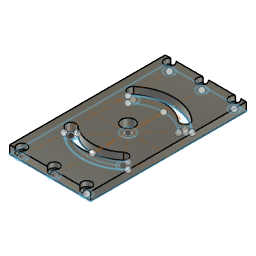
FS80 Pivot Base v3 (Autodesk Fusion 360 design; units mm, degrees)
Autodesk Fusion 360 part; units mm, degrees
sketch "Schizzo5" plane through (0, 0, 0) normal (0, 0, 1) x (1, 0, 0)
  line L0 (80.7173, 86.3147) -> (80.7173, -9.6853)
  circle A0 centre (85.7173, -7.1853) radius 1.5
  circle A1 centre (105.7173, 38.3147) radius 25 construction
  arc A2 (125.5163, 58.1137) -> (105.7173, 66.3147) centre (105.7173, 38.3147) ccw
  circle A3 centre (121.787, 57.4658) radius 3
  circle A4 centre (89.6476, 57.4658) radius 3
  arc A5 (105.7173, 66.3147) -> (85.9183, 58.1137) centre (105.7173, 38.3147) ccw
  circle A6 centre (125.7173, 83.8147) radius 3
  arc A7 (105.7173, 10.3147) -> (125.5163, 18.5157) centre (105.7173, 38.3147) ccw
  line L1 (80.7173, 38.3147) -> (130.7173, 38.3147) construction
  circle A8 centre (105.7173, 83.8147) radius 1.5
  circle A9 centre (85.7173, 83.8147) radius 3
  line L2 (105.7173, 38.3147) -> (121.787, 19.1636) construction
  arc A10 (105.7173, 66.3147) -> (85.9183, 58.1137) centre (105.7173, 38.3147) ccw
  circle A11 centre (85.7173, 83.8147) radius 1.5
  line L3 (130.7173, 86.3147) -> (80.7173, 86.3147)
  arc A12 (125.5163, 58.1137) -> (105.7173, 66.3147) centre (105.7173, 38.3147) ccw
  circle A13 centre (125.7173, 83.8147) radius 1.5
  line L4 (105.7173, 38.3147) -> (89.6274, 54.4047) construction
  circle A14 centre (105.7173, 83.8147) radius 3
  arc A15 (105.7173, 10.3147) -> (125.5163, 18.5157) centre (105.7173, 38.3147) ccw
  line L5 (105.7173, 38.3147) -> (105.7173, 13.3147) construction
  circle A16 centre (105.7173, 38.3147) radius 4.1
  circle A17 centre (105.7173, -7.1853) radius 1.5
  circle A18 centre (89.6476, 19.1636) radius 3
  line L6 (130.7173, -9.6853) -> (130.7173, 86.3147)
  arc A19 (85.9183, 18.5157) -> (105.7173, 10.3147) centre (105.7173, 38.3147) ccw
  line L7 (85.7173, 86.3147) -> (85.7173, -9.6853) construction
  arc A20 (105.7173, 13.3147) -> (121.787, 19.1636) centre (105.7173, 38.3147) ccw
  circle A21 centre (121.787, 19.1636) radius 3
  circle A22 centre (85.7173, -7.1853) radius 3
  circle A23 centre (105.7173, -7.1853) radius 3
  circle A24 centre (125.7173, -7.1853) radius 1.5
  line L8 (105.7173, 38.3147) -> (123.668, 56.2654) construction
  line L9 (80.7173, -9.6853) -> (130.7173, -9.6853)
  circle A25 centre (125.7173, -7.1853) radius 3
  line L10 (80.7173, -7.1853) -> (130.7173, -7.1853) construction
  line L11 (105.7173, 38.3147) -> (89.6476, 19.1636) construction
  arc A26 (85.9183, 18.5157) -> (105.7173, 10.3147) centre (105.7173, 38.3147) ccw
  line L12 (105.7173, 86.3147) -> (105.7173, -9.6853) construction
  arc A27 (89.6476, 19.1636) -> (105.7173, 13.3147) centre (105.7173, 38.3147) ccw
  line L13 (105.7173, 38.3147) -> (105.7173, 63.3147) construction
  line L14 (105.7173, 38.3147) -> (105.7173, 63.3147) construction
  line L15 (105.7173, 38.3147) -> (105.7173, 13.3147) construction
  arc A28 (105.7173, 16.3147) -> (121.2737, 22.7584) centre (105.7173, 38.3147) ccw
  arc A29 (90.161, 22.7584) -> (105.7173, 16.3147) centre (105.7173, 38.3147) ccw
  arc A30 (105.7173, 60.3147) -> (90.161, 53.8711) centre (105.7173, 38.3147) ccw
  arc A31 (121.2737, 53.8711) -> (105.7173, 60.3147) centre (105.7173, 38.3147) ccw
  dimension "d219" = 3
  dimension "d220" = 3
  dimension "d221" = 50
  dimension "d222" = 96
  dimension "d223" = 2.5
  dimension "d224" = 20
  dimension "d225" = 3
  dimension "d226" = 6
  dimension "d227" = 3
  dimension "d228" = 6
  dimension "d229" = 8.2
  dimension "d230" = 40
  dimension "d231" = 6
  dimension "d232" = 40
  dimension "d233" = 6
  dimension "d246" = -3
  dimension "d247" = -3
  constraint horizontal L9
  constraint vertical L6
  constraint horizontal L3
  constraint vertical L0
  constraint midpoint L12.start L3
  constraint midpoint L12.end L9
  constraint coincident L10.end L6
  constraint perpendicular L6 L10
  constraint midpoint L1.start L0
  constraint midpoint L1.end L6
  constraint coincident L7.start L3
  constraint coincident L7.end L9
  constraint perpendicular L7 L9
  constraint coincident A0.centre L10
  constraint coincident A0.centre L7
  constraint concentric A0 A22
  constraint symmetric A0 A24 L12
  constraint symmetric A22 A25 L12
  constraint symmetric A0 L1 A11
  constraint symmetric L1 A9 A22
  constraint symmetric L1 A13 A24
  constraint symmetric A6 L1 A25
  constraint coincident A17.centre L12
  constraint coincident A17.centre L10
  constraint concentric A17 A23
  constraint symmetric L1 A8 A17
  constraint symmetric L1 A14 A23
  constraint midpoint A1.centre L1
  constraint concentric A1 A16
  constraint tangent A1 L6
  constraint coincident L5.end A1
  constraint coincident L5.end L12
  constraint coincident A1.centre A2.centre
  constraint coincident A18.centre L11.end
  constraint coincident L2.end A20.end
  constraint coincident L13.end A1
  constraint coincident L13.end L12
  constraint symmetric A4 L1 A18
  constraint symmetric A3 L1 A21
  constraint symmetric A7.start A2.end L1
  constraint symmetric A19.start A5.end L1
  constraint symmetric A5 L1 A19
  constraint symmetric A7.end A2.start L1
  constraint symmetric A2 L1 A15
  constraint symmetric A5.end A19.start L1
  constraint symmetric L1 A10 A26
  constraint symmetric A7 L1 A12
  constraint symmetric L1 A28.end A31.start
  constraint symmetric L1 A28.start A30.start
  constraint symmetric L1 A28 A31
  constraint symmetric L1 A29.start A30.end
  constraint symmetric L1 A29 A30
  constraint coincident L10.start L0
  measures "d221" distance of L0.end L6.start
  measures "d222" distance of L0.end L0.start
  measures "d223" distance of L9 L10
  measures "d224" distance of L7 L12
  measures "d225" diameter of A0
  measures "d226" diameter of A22
  measures "d227" diameter of A17
  measures "d228" diameter of A23
  measures "d229" diameter of A16
  measures "d230" angle of L11 L15
  measures "d231" diameter of A18
  measures "d232" angle of L2 L5
  measures "d233" diameter of A21
extrude "Estrusione24" add sketch "Schizzo5" along normal blind 5 contours L0 A6 A9 L3 A14 L6 A22 A23 L9 A25
extrude "Estrusione25" add sketch "Schizzo5" along normal blind 1.8 contours A9 L3 | A22 L9 | L3 A14 | A23 L9 | A6 L3 | L9 A25 picked at (85.7547, 85.98) picked at (85.7547, -9.3505) picked at (105.7547, 85.98) picked at (105.7547, -9.3505) picked at (125.7547, 85.98) picked at (125.7547, -9.3505)
equation "d225 = d227"
equation "d226 = d228"
named bodies: "Base"
